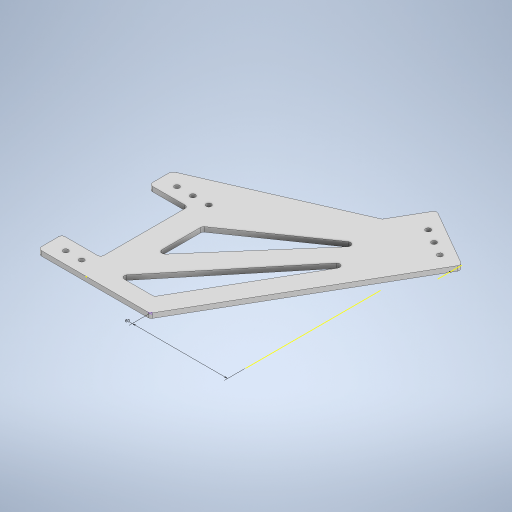
# Autodesk Inventor part: オムニ_前2_N
Saved by Autodesk Inventor 2023 (Build 270158000, 158)
## iProperties
Created: 2022-04-13
Part Number: オムニ_前2_N
Material: Generic
Document SubType Name: Sheet Metal
Designer: yuta
Density: 1 g/cm^3
Sheet Metal Rule: Default
Appearance: Default
Author: yuta
Autodesk Inventor part; units mm, degrees
ref_plane "YZ Plane" through (0, 0, 0) normal (1, 0, 0) x (0, 1, 0)
ref_plane "XZ Plane" through (0, 0, 0) normal (0, 1, 0) x (-1, 0, 0)
ref_plane "XY Plane" through (0, 0, 0) normal (0, 0, 1) x (1, 0, 0)
sketch "スケッチ1" plane through (0, 0, 0) normal (0, 1, 0) x (-1, 0, 0)
  line L0 (0, 0) -> (30.5, 0)
  line L1 (30.5, 0) -> (30.5, -85)
  line L2 (30.5, -85) -> (0, -85)
  line L3 (0, -85) -> (0, 0)
  dimension "d0" = 30.5
  dimension "d1" = 85
  constraints: 8 end point, 2 parallel, 1 horizontal, 1 perpendicular
  measures "d0" distance of L1.end L2.end
  measures "d1" distance of L0.end L1.end
extrude "押し出し1" add sketch "スケッチ1" along normal blind 3
sketch "スケッチ2" plane through (0, 3, 0) normal (0, 1, 0) x (1, 0, 0)
  line L0 (-30.5464, 15) -> (-6.0464, 15)
  line L1 (-6.0464, 15) -> (-6.0464, 70)
  line L2 (-6.0464, 70) -> (-30.5464, 70)
  line L3 (-30.5, 0) -> (0, 0) projected
  line L4 (-30.5464, 15) -> (-30.5464, 70)
  dimension "d4" = 24.5
  dimension "d5" = 55
  dimension "d6" = 90
  dimension "d7" = 15
  constraints: 8 end point, 3 perpendicular, 1 horizontal
  measures "d4" distance of L0.start L0.end
  measures "d5" distance of L0.end L1.end
  measures "d6" angle of L1 L0
  measures "d7" distance between parallel lines of L3 L0
extrude "押し出し2" cut sketch "スケッチ2" against normal blind 3
fillet "フィレット1" radius 2 4 edges at (-30.5, 1.5, 0) (-30.5, 1.5, -70) (-30.5, 1.5, -85) (-30.5, 1.5, -15)
fillet "フィレット2" radius 2 2 edges at (-6.0464, 1.5, -15) (-6.0464, 1.5, -70)
sketch "スケッチ3" plane through (0, 3, 0) normal (0, 1, 0) x (1, 0, 0)
  line L0 (-28.5, 0) -> (0, 0) projected
  line L1 (0, 0) -> (100, 0)
  line L2 (100, 0) -> (100, 85)
  line L3 (100, 85) -> (0, 85)
  line L4 (0, 85) -> (0, 0)
  dimension "d12" = 100
  dimension "d13" = 85
  constraints: 8 end point, 2 parallel, 1 horizontal, 1 perpendicular
  measures "d12" distance of L3.end L2.end
  measures "d13" distance of L2.end L1.end
extrude "押し出し3" add sketch "スケッチ3" against normal blind 3
sketch "スケッチ4" plane through (0, 3, 0) normal (0, 1, 0) x (1, 0, 0)
  line L0 (100, 0) -> (100, 85) projected
  point P0 (0, 0)
  point P1 (40, 0)
  dimension "d16" = 60
  measures "d16" distance from line of point (40, 0) L0
sketch "スケッチ5" plane through (0, 3, 0) normal (0, 1, 0) x (1, 0, 0)
  line L0 (-28.5, 0) -> (100, 0) projected
  line L1 (39.9909, 0) -> (111.8004, 124.3777)
  line L2 (39.9909, 0) -> (183.6099, 0) construction
  line L3 (111.8004, 124.3777) -> (61.8004, 124.3777)
  line L4 (61.8004, 124.3777) -> (-28.5, 85)
  line L5 (-28.5, 85) -> (89.0656, 85)
  line L6 (100, 85) -> (-28.5, 85) projected
  point P0 (0, 0)
  dimension "d17" = 143.619
  dimension "d18" = 60
  dimension "d19" = 50
  constraints: 10 end point, 3 point on line, 1 equal length, 1 horizontal, 1 parallel
  measures "d17" distance of L1.start L1.end
  measures "d18" angle of L2 L1
  measures "d19" distance of L1.end L3.end
extrude "押し出し4" add sketch "スケッチ5" against normal blind 3
sketch "スケッチ6" plane through (0, 3, 0) normal (0, 1, 0) x (1, 0, 0)
  line L0 (111.8004, 124.3777) -> (61.8004, 124.3777) projected
  line L1 (111.8004, 124.3777) -> (111.8004, 0)
  line L2 (111.8004, 124.3777) -> (236.1781, 124.3777) construction
  line L3 (100, 0) -> (100, 85) projected
  line L4 (111.8004, 0) -> (100, 0)
  line L5 (100, 0) -> (100, 85)
  line L6 (100, 85) -> (89.0656, 85) projected
  line L7 (100, 85) -> (89.0656, 85)
  line L8 (89.0656, 85) -> (111.8004, 124.3777) projected
  line L9 (89.0656, 85) -> (111.8004, 124.3777)
  point P0 (0, 0)
  dimension "d22" = 90
  constraints: 12 end point, 3 perpendicular, 2 collinear, 1 horizontal
  measures "d22" angle of L1 L2
extrude "押し出し5" add sketch "スケッチ6" against normal blind 3
sketch "スケッチ7" plane through (0, 3, 0) normal (0, 1, 0) x (1, 0, 0)
  line L0 (111.8004, 124.3777) -> (111.8004, 0) projected
  line L1 (111.8004, 109.3777) -> (39.991, 0)
  line L2 (-28.5, 0) -> (111.8004, 0) projected
  line L3 (111.8004, 0) -> (111.8004, 109.3777)
  line L4 (111.8004, 0) -> (39.991, 0)
  point P0 (0, 0)
  dimension "d25" = 15
  constraints: 6 end point, 2 point on line, 1 perpendicular
  measures "d25" distance of L0.start L1.start
extrude "押し出し6" cut sketch "スケッチ7" against normal blind 3
sketch "スケッチ8" plane through (0, 3, 0) normal (0, 1, 0) x (1, 0, 0)
  line L0 (111.8004, 109.3777) -> (111.8004, 124.3777) projected
  point P0 (0, 0)
  point P1 (111.8004, 116.8777)
  constraints: 1 midpoint
sketch "スケッチ9" plane through (0, 3, 0) normal (0, 1, 0) x (1, 0, 0)
  point P0 (0, 0)
sketch "スケッチ10" plane through (0, 3, 0) normal (0, 1, 0) x (1, 0, 0)
  line L0 (111.8004, 109.3777) -> (39.991, 0) projected
  line L1 (61.8004, 124.3777) -> (111.8004, 124.3777) projected
  line L2 (39.991, 0) -> (111.8004, 124.3777)
  line L3 (111.8004, 109.3777) -> (111.8004, 124.3777) projected
  line L4 (111.8004, 124.3777) -> (111.8004, 109.3777)
  line L5 (111.8004, 109.3777) -> (39.991, 0)
  point P0 (0, 0)
  constraints: 6 end point, 1 collinear
extrude "押し出し7" cut sketch "スケッチ10" against normal blind 3
sketch "スケッチ11" plane through (0, 3, 0) normal (0, 1, 0) x (1, 0, 0)
  line L0 (61.8004, 124.3777) -> (74.3769, 146.1608)
  line L1 (61.8004, 124.3777) -> (86.9534, 124.3777) construction
  line L2 (74.3769, 146.1608) -> (112.1064, 124.3777)
  line L3 (111.8004, 124.3777) -> (61.8004, 124.3777) projected
  line L4 (112.1064, 124.3777) -> (61.8004, 124.3777)
  point P0 (0, 0)
  dimension "d32" = 25.153
  dimension "d33" = 60
  constraints: 8 end point, 1 collinear, 1 equal length, 1 horizontal, 1 perpendicular
  measures "d32" distance of L0.start L0.end
  measures "d33" angle of L1 L0
extrude "押し出し8" add sketch "スケッチ11" against normal blind 3
fillet "フィレット3" radius 2 2 edges at (112.1064, 1.5, -124.3777) (111.8004, 1.5, -124.3777)
fillet "フィレット4" radius 2 3 edges at (74.3769, 1.5, -146.1608) (61.8004, 1.5, -124.3777) (39.991, 1.5, 0)
sketch "スケッチ12" plane through (0, 3, 0) normal (0, 1, 0) x (1, 0, 0)
  circle A0 centre (99.4666, 123.015) radius 1.6
  line L0 (110.1448, 125.5102) -> (76.1089, 145.1608) projected
  line L1 (40.5683, 1) -> (110.8769, 122.7782) projected
  circle A1 centre (89.4666, 128.7885) radius 1.6
  circle A2 centre (79.4666, 134.562) radius 1.6
  point P0 (0, 0)
  dimension "d38" = 3.2
  dimension "d39" = 7.5
  dimension "d40" = 10
  dimension "d41" = 3.2
  dimension "d42" = 3.2
  dimension "d43" = 10
  dimension "d44" = 7.5
  dimension "d45" = 7.5
  dimension "d46" = 10
  constraints: 3 centre point
  measures "d38" diameter of A0
  measures "d39" distance from line of L0 A0.centre
  measures "d40" distance from line of L1 A0.centre
  measures "d41" diameter of A1
  measures "d42" diameter of A2
  measures "d43" horizontal distance of A0.centre A1.centre
  measures "d44" distance from line of L0 A1.centre
  measures "d45" distance from line of L0 A2.centre
  measures "d46" horizontal distance of A1.centre A2.centre
hole "穴1" at (99.4666, 3, -123.015) at (89.4666, 3, -128.7885) at (79.4666, 3, -134.562) direction (0, -1, 0) diameter 3.2 depth 3.048
fillet "フィレット5" radius 2 1 edges at (-28.5, 1.5, -85)
sketch "スケッチ13" plane through (0, 3, 0) normal (0, 1, 0) x (1, 0, 0)
  line L0 (-30.5, 83) -> (-30.5, 72) projected
  line L1 (-28.1853, 85.1373) -> (61.1969, 124.1146) projected
  line L2 (-30.5, 83) -> (-28.1853, 85.1373)
  line L3 (-28.1853, 85.1373) -> (-30.5, 84.8107)
  arc A0 (-28.7424, 84.9853) -> (-30.5, 83) centre (-28.5, 83) ccw projected
  line L4 (-30.5, 84.8107) -> (-30.5, 83)
  point P0 (0, 0)
  constraints: 6 end point, 1 tangent, 1 vertical
extrude "押し出し9" cut sketch "スケッチ13" against normal blind 3
fillet "フィレット6" radius 2 2 edges at (-28.1853, 1.5, -85.1373) (-30.5, 1.5, -83)
sketch "スケッチ14" plane through (0, 3, 0) normal (0, 1, 0) x (1, 0, 0)
  circle A0 centre (-20.5, 77.5) radius 1.6
  line L0 (-30.5, 82.1245) -> (-30.5, 72) projected
  line L1 (-28.5, 70) -> (-8.0464, 70) projected
  circle A1 centre (-10.5, 77.5) radius 1.6
  circle A2 centre (-0.5, 77.5) radius 1.6
  circle A3 centre (-20.5, 7.5) radius 1.6
  line L2 (-8.0464, 15) -> (-28.5, 15) projected
  line L3 (-30.5, 13) -> (-30.5, 2) projected
  circle A4 centre (-10.5, 7.5) radius 1.6
  point P0 (0, 0)
  dimension "d58" = 3.2
  dimension "d59" = 10
  dimension "d60" = 7.5
  dimension "d61" = 3.2
  dimension "d62" = 3.2
  dimension "d63" = 10
  dimension "d64" = 7.5
  dimension "d65" = 10
  dimension "d66" = 7.5
  dimension "d67" = 3.2
  dimension "d68" = 7.5
  dimension "d69" = 10
  dimension "d70" = 3.2
  dimension "d71" = 10
  dimension "d72" = 7.5
  constraints: 5 centre point
  measures "d58" diameter of A0
  measures "d59" distance from line of L0 A0.centre
  measures "d60" distance from line of L1 A0.centre
  measures "d61" diameter of A1
  measures "d62" diameter of A2
  measures "d63" distance of A1.centre A0.centre
  measures "d64" distance from line of L1 A1.centre
  measures "d65" distance of A1.centre A2.centre
  measures "d66" distance from line of L1 A2.centre
  measures "d67" diameter of A3
  measures "d68" distance from line of L2 A3.centre
  measures "d69" distance from line of L3 A3.centre
  measures "d70" diameter of A4
  measures "d71" distance of A3.centre A4.centre
  measures "d72" distance from line of L2 A4.centre
hole "穴2" at (-20.5, 3, -7.5) at (-10.5, 3, -7.5) at (-20.5, 3, -77.5) at (-10.5, 3, -77.5) at (-0.5, 3, -77.5) direction (0, -1, 0) diameter 3.2 depth 3.048
sketch "スケッチ15" plane through (0, 3, 0) normal (0, 1, 0) x (1, 0, 0)
  line L0 (32.1999, 10.4234) -> (86.628, 104.6956)
  line L1 (32.1999, 10.4234) -> (141.0561, 10.4234) construction
  line L2 (86.628, 104.6956) -> (9.117, 10.4234)
  line L3 (9.117, 10.4234) -> (32.1999, 10.4234)
  line L4 (9.117, 33.0287) -> (76.4814, 110.5538)
  line L5 (76.4814, 110.5538) -> (9.117, 63.797)
  line L6 (9.117, 63.797) -> (9.117, 33.0287)
  point P0 (0, 0)
  dimension "d80" = 60
  constraints: 14 end point, 2 horizontal, 1 equal length, 1 perpendicular, 1 point on line
  measures "d80" angle of L1 L0
extrude "押し出し10" cut sketch "スケッチ15" against normal blind 3
fillet "フィレット7" radius 2 6 edges at (9.117, 1.5, -63.797) (9.117, 1.5, -10.4234) (32.1999, 1.5, -10.4234) (9.117, 1.5, -33.0287) (76.4814, 1.5, -110.5538) (86.628, 1.5, -104.6956)
sketch "スケッチ16" plane through (0, 3, 0) normal (0, 1, 0) x (1, 0, 0)
  circle A0 centre (99.4666, 123.015) radius 1.6 projected
  circle A1 centre (99.4666, 123.015) radius 1.6
  circle A2 centre (89.4666, 128.7885) radius 1.6 projected
  circle A3 centre (89.4666, 128.7885) radius 1.6
  circle A4 centre (79.4666, 134.562) radius 1.6 projected
  circle A5 centre (79.4666, 134.562) radius 1.6
  point P0 (0, 0)
  dimension "d84" = 3.2
  dimension "d85" = 3.2
  dimension "d86" = 3.2
  constraints: 3 centre point, 3 coincident
  measures "d84" diameter of A1
  measures "d85" diameter of A3
  measures "d86" diameter of A5
extrude "押し出し11" add sketch "スケッチ16" against normal blind 3
sketch "スケッチ17" plane through (0, 3, 0) normal (0, 1, 0) x (1, 0, 0)
  circle A0 centre (99.4666, 123.015) radius 1.6
  line L0 (110.1448, 125.5102) -> (76.1089, 145.1608) projected
  line L1 (40.5683, 1) -> (110.8769, 122.7782) projected
  circle A1 centre (90.8064, 128.015) radius 1.6
  circle A2 centre (82.1461, 133.015) radius 1.6
  point P0 (0, 0)
  dimension "d89" = 3.2
  dimension "d90" = 7.5
  dimension "d91" = 10
  dimension "d92" = 3.2
  dimension "d93" = 3.2
  dimension "d95" = 7.5
  dimension "d97" = 7.5
  dimension "d98" = 20
  dimension "d99" = 30
  constraints: 3 centre point
  measures "d89" diameter of A0
  measures "d90" distance from line of L0 A0.centre
  measures "d91" distance from line of L1 A0.centre
  measures "d92" diameter of A1
  measures "d93" diameter of A2
  measures "d95" distance from line of L0 A1.centre
  measures "d97" distance from line of L0 A2.centre
  measures "d98" distance from line of L1 A1.centre
  measures "d99" distance from line of L1 A2.centre
hole "穴3" at (82.1461, 3, -133.015) at (90.8064, 3, -128.015) at (99.4666, 3, -123.015) direction (0, -1, 0) diameter 3.2 depth 3.048
equation "\"d52\" = Thickness"
equation "\"d78\" = Thickness"
equation "\"d105\" = Thickness"
equation "\"BendRadius\" = Thickness"
equation "\"BendReliefWidth\" = Thickness"
equation "\"BendReliefDepth\" = 0.5 * Thickness"
equation "\"CornerReliefSize\" = 4 * Thickness"
equation "\"MinimumRemnant\" = 2 * Thickness"
equation "\"TransitionRadius\" = BendRadius"
equation "\"JacobiRadiusSize\" = BendRadius"
equation "\"GapSize\" = Thickness"
equation "\"Thickness\" = 3.048"
